Autodesk Fusion 360 part; units mm, degrees
(part 2 of 2)
extrude "Extrude1" add sketch "Sketch1" along normal blind 1.7 contours L0 L26 L52 L57 L77 L124 L128 L191 | L0 L12 L33 L120 L124 L128 L189 L191 | L0 L26 L33 L36 L52 L124 L128 L191 | L0 L12 L57 L120 L121 L124 L125 L128 L189 L191 | L0 L26 L57 L74 L76 L77 L191 L207 A39 | L0 L12 L57 L74 L121 L125 L126 L189 L191 L217 | L0 L12 L29 L32 L33 L189 L191 | L0 L26 L29 L33 L36 L191 | L26 L52 L57 L124 L127 L128 L220 | L26 L37 L52 L124 L128 L221 | L0 L26 L75 L78 L126 L191 L207 L217 L218 | L26 L75 L76 L78 L207 A39 | L26 L57 L76 L208 A39 | L0 L12 L28 L29 L32 A15 L189 L191 | L0 L26 L29 L36 A16 L191 | L26 L27 L33 L34 L36 L37 L39 L42 A26 L287 | L26 L27 L33 L34 A1 L36 L39 A26 | L52 L57 L123 L124 L127 | L0 L26 L122 L126 L191 L207 L218 | L0 L12 L121 L122 L126 L189 L191 | L26 L78 L207 A38 | L26 L76 L78 L207 L208 A38 A39 | L26 L76 L207 L208 A39 | L57 L127 L208 L219 L220 A39 | L3 L13 L26 L27 L30 L31 L35 L36 L39 A15 A16 L191 | L29 L30 A0 A1 | L26 L27 A1 L36 L39 A16 | L29 L30 A0 A1 | L27 L37 L39 L41 L42 L43 L287 L288 L289 L290 L291 L292 | L37 L41 L47 L52 L64 L109 L115 L119 L221 L288 | L52 L57 L123 L221 | L57 L123 L127 L208 L219 | L0 L26 L122 L130 L191 L193 L199 L207 | L0 L12 L122 L189 L191 L198 | L26 L78 L122 L123 A27 L207 A38 | L78 L126 A7 A38 L218 | L78 L126 A7 A38 L218 | L78 L127 A7 A38 L219 | L26 L27 L36 L39 A16 | L29 L30 A0 | L29 L30 A0 | L3 L27 L30 L34 L39 | L3 L27 L30 L39 A16 | L37 L40 L41 L44 L289 L293 | L3 L27 L34 L39 L43 L45 A25 L290 | L52 L57 L82 L114 L178 L221 | L57 L79 L123 L208 L221 | L78 L127 A7 A38 L219 | L78 L123 L208 A38 | L0 L12 L189 L191 L196 L197 L198 L199 | L25 L26 L78 L80 L83 L122 L123 L130 L131 A27 A28 L206 L207 L223 L224 L226 L230 L234 L237 | L78 L126 L127 A7 L218 L219 | L78 L126 L127 A7 L218 L219 | L78 L127 A7 L219 | L3 L13 L30 L34 L35 | L27 L37 L39 L40 L44 L45 L46 L47 L293 L294 L295 | L40 L44 L289 L291 L292 L293 L295 | L27 L39 L40 L43 L44 L289 L295 | L52 L57 L114 L115 L118 L212 | L57 L79 L81 L82 L208 L221 | L78 L79 L123 L208 L221 | L78 L127 A7 L219 | L0 L12 L189 L191 L193 L194 L195 L196 L197 L199 L200 | L25 L26 L130 L131 A9 A28 L206 L207 | L0 L26 L130 L134 L191 L207 | L3 L4 L13 L18 L19 L27 L34 L39 A24 A25 | L24 L27 L37 L38 L39 L46 L63 L64 L66 A23 A25 | L40 L44 L293 L294 L295 | L52 L57 L108 L115 L118 L119 L204 L212 | L57 L91 L114 L177 L208 L211 | L57 L91 L114 L118 L208 L211 L212 L216 | L57 L81 L179 L208 | L78 L79 L80 L81 L208 L221 | L0 L12 L130 L189 L191 L194 L200 | L25 L26 A9 A18 L206 L207 | L0 L26 L134 A18 L191 L207 | L134 L135 A8 A9 | L134 L135 A8 A9 | L0 L12 L129 L130 L134 L189 L191 | L24 L37 L38 L63 L64 A3 A23 | L37 L52 L60 L64 L181 | L52 L57 L108 L109 L110 L112 L115 L116 L119 | L57 L118 L208 L212 A36 | L57 L177 L178 L179 L208 | L78 L91 L114 L118 A6 L208 L211 L215 L216 | L78 L91 L114 L177 L208 L211 L215 | L78 L81 L86 L179 L208 | L25 L26 A18 L206 L207 | L21 L26 A18 L191 L207 | L0 L11 L12 L20 L129 L133 L134 A17 L189 L191 | L134 L135 A8 | L134 L135 A8 | L1 L25 L135 A18 L206 | L1 L25 L131 L135 L206 | L24 L27 L38 L39 A25 | L24 L37 L38 A3 A22 | L59 L60 A2 A3 L181 L184 | L37 L52 L60 L181 L182 A22 | L59 L60 A2 A3 L181 L184 | L52 L57 L64 L110 L112 L116 | L52 L57 L60 L64 L65 | L57 L108 L201 L202 L203 L204 | L57 L78 L108 L110 L112 L116 L201 | L57 L203 L208 A36 | L78 L118 A6 A37 | L78 L205 L208 A36 A37 | L78 L86 L177 L179 L208 | L78 L85 L91 L114 L170 L176 L177 L211 L215 | L78 L91 L113 L114 L117 A6 A29 L205 L210 L211 L213 L214 L215 | L78 L83 L86 L138 L139 L161 L164 L179 L222 L223 L238 L241 L250 | L20 L21 L22 L23 L191 | L1 L8 L15 L22 L23 L25 L132 L135 L136 A17 A18 L191 L206 | L1 L25 L131 L206 L230 | L1 L15 L131 L132 L135 | L4 L7 A24 | L16 L17 L18 L19 | L2 L7 L14 L16 L17 L24 L38 L71 A24 A25 | L2 L24 L38 L69 L70 A25 | L24 L37 L38 A22 | L24 L37 L48 L52 A22 | L59 L60 A2 L181 L184 | L59 L60 A2 L181 L184 | L24 L52 L57 L60 L61 L65 A21 L182 | L2 L24 L38 L59 L183 L184 A22 | L2 L24 L38 L59 L63 L184 | L108 L202 L205 A36 | L205 L208 A36 | L78 L118 A6 | L78 L118 A6 | L78 L117 A6 A37 | L78 L205 A37 | L78 L85 L86 L138 L176 L177 L179 L180 A32 L254 | L78 L117 L118 A6 | L91 A29 L210 L211 L214 L215 | L25 L83 L84 L206 L222 L223 L225 A44 L247 L248 A46 | L25 L83 L206 L223 L224 L225 L231 L232 A42 A47 A48 | L25 L206 L224 L225 L226 L227 L228 L229 A40 L230 | L1 L25 L206 L225 L229 L230 L232 L233 | L1 L15 L88 L92 L102 L131 L144 L154 L160 L233 L249 | L2 L24 L38 L66 L67 L69 | L2 L24 L48 L49 L50 L51 L52 | L2 L24 L38 L51 A22 | L2 L24 L38 L63 L67 | L2 L14 L50 L56 L58 L59 L62 A21 L183 | L2 L14 L59 L62 L63 | L78 L108 L110 L112 L116 L117 L209 | L78 L108 L117 L205 L209 | L78 L205 A36 | L78 L117 L118 A6 | L108 L113 L117 L205 L209 L210 L213 | L85 L91 L137 L165 L169 L170 L171 L172 L173 L176 L177 L251 | L85 L138 L168 L169 L176 L177 L180 A32 L254 | L91 L101 L113 L171 L173 L188 L205 L210 L214 | L25 L84 L85 L137 L138 L139 L140 L142 L143 L158 L159 A14 L180 A30 A34 L206 L250 L252 L253 L283 L284 L285 L286 A63 A64 A65 | L1 L25 L84 L206 L225 L232 L248 | L239 L240 A43 A44 | L222 L223 L238 L241 A44 | L239 L240 A43 A44 | L223 L224 L234 L237 A42 | L235 L236 A41 A42 | L235 L236 A41 A42 | L8 L11 A17 L191 | L25 L206 L224 L225 L227 L228 A40 L230 L231 L232 A47 A48 | L2 L14 L67 L68 L69 L73 | L2 L14 L69 L70 L71 L72 L73 | L2 L24 L49 L52 L53 A21 | L2 L14 L63 L67 | L108 L110 L112 L113 L117 L209 | L101 L108 L113 L205 L210 | L85 L137 L138 L165 L168 L169 L180 L251 L254 A66 | L138 L175 L180 A32 L253 L254 L280 L286 | L138 L139 L161 L164 A14 | L162 L163 A12 A14 | L162 L163 A12 A14 | L25 L84 L157 L206 L222 L225 L243 L244 A45 L246 L247 L248 A46 | L1 L25 L84 L155 L157 L206 L225 L245 L246 L248 L249 | L239 L240 A43 | L239 L240 A43 | L235 L236 A41 | L235 L236 A41 | L227 L228 A40 | L227 L228 A40 | L1 L15 L92 L93 L95 L102 L103 L106 | L2 L53 L56 A21 | L101 L108 L110 L113 | L101 A5 A31 L205 | L101 L105 L108 L205 | L85 L91 L137 L172 L173 L174 L251 | L166 L167 A13 A66 | L85 L137 L138 L174 L175 L180 A32 A33 L251 L254 L280 L281 L283 A66 | L166 L167 A13 A66 | L175 A33 L252 L253 L271 L272 L273 L274 L275 L278 L279 L280 L281 L282 L283 L286 A61 A62 | L252 L253 L275 L276 L277 L278 L279 L282 L283 L284 L285 L286 A56 A57 A59 A63 A64 A65 | L162 L163 A12 | L162 L163 A12 | L25 L84 L157 L206 L222 L225 L242 L243 L244 L245 A45 L246 | L139 A35 L222 L246 L250 | L1 L15 L93 L95 L98 L103 L106 L107 A19 | L1 L25 L89 L91 L95 L102 L106 L141 L206 | L1 L25 L87 L88 L89 L90 L91 L102 L141 L144 L206 | L100 L101 L105 L108 L110 | L91 L101 L102 L141 L185 L188 A31 | A5 L187 A31 | A5 L186 L187 A31 | L105 L106 A4 A5 | L25 A5 A20 L205 L206 | L105 A4 A5 A31 | L105 L108 A20 L205 | L85 L91 L137 L142 L174 L251 | L85 L137 L174 A33 L251 L252 L281 L283 | L166 L167 A13 | L166 L167 A13 | L253 L264 L270 L271 L278 L279 A61 | L252 L253 L267 L268 L269 L270 L275 L276 L277 L278 L279 L282 A54 A55 A56 A57 A58 A59 | L175 L280 A62 | L139 A35 L250 | L25 L84 L139 L149 L156 L157 A35 L206 L222 L242 L246 | L1 L25 L84 L140 L152 L153 L154 L155 L156 L157 L160 L206 L246 | L243 L244 A45 | L243 L244 A45 | L1 L25 L95 L106 A20 L206 | L1 L25 L84 L87 L140 L143 L144 L148 L206 | L25 L91 L102 A5 L141 A31 L206 | L25 L85 L90 L91 L102 L137 L141 L142 L145 L185 L206 | L25 L95 L97 A19 A20 L206 | L25 L100 L104 L105 L108 L110 A19 A20 L205 | A5 L186 L187 | A4 A5 L186 L187 A31 | A5 L186 A31 | L105 L106 A4 | L105 L106 A4 A31 | L106 A4 A5 A31 | L25 A20 L205 L206 | L175 L280 L281 A62 | L252 L253 L256 L257 L259 L262 L263 L264 L265 L266 L267 L270 L279 L282 A60 | L252 L253 L259 L260 L261 L262 L263 L266 L267 L268 L269 L270 L279 L282 A50 A51 A52 A54 A55 A58 | L175 A33 L281 L283 A62 | L25 L84 L139 L140 L150 L151 A11 L158 L159 A34 A35 L206 L250 | L25 L84 L139 L140 L149 L150 L151 L152 A11 L156 L206 | L1 L25 L84 L140 L153 L159 L160 L206 | L95 L97 L98 A19 | L1 L25 L84 L140 L143 L159 L206 | L25 L84 L85 L137 L140 L145 L146 L147 L148 A10 L206 | L25 L84 L85 L137 L140 L142 L143 L146 L147 A10 A30 L206 | A4 A31 | L252 L253 A49 L255 L256 L257 L258 L259 L262 L263 L266 L279 L282 A53 | L252 L253 A49 L255 L258 L259 L260 L261 L262 L263 L266 L279 L282 A50 A51 A52 | L264 L265 A60 | L271 L274 A61 | L271 L272 L273 L274 A61 | L252 L265 L267 L274 L275 L282 A61 | L252 L253 A49 L255 L258 L263 L266 L279 L282 | L252 L253 A49 L255 L258 L263 L266 L279 L282 | L256 L257 A53 | L150 L151 A11 | L150 L151 A11 | L146 L147 A10 | L146 L147 A10 makes body 1
extrude "Extrude2" add sketch "Sketch1" along normal blind 13.7 contours L0 L12 L33 L120 L124 L128 L189 L191 | L0 L12 L57 L120 L121 L124 L125 L128 L189 L191 | L0 L12 L57 L74 L121 L125 L126 L189 L191 L217 | L0 L12 L29 L32 L33 L189 L191 | L0 L12 L28 L29 L32 A15 L189 L191 | L0 L12 L121 L122 L126 L189 L191 | L3 L13 L26 L27 L30 L31 L35 L36 L39 A15 A16 L191 | L0 L12 L122 L189 L191 L198 | L26 L27 L36 L39 A16 | L0 L12 L189 L191 L196 L197 L198 L199 | L3 L13 L30 L34 L35 | L0 L12 L189 L191 L193 L194 L195 L196 L197 L199 L200 | L3 L4 L13 L18 L19 L27 L34 L39 A24 A25 | L0 L12 L130 L189 L191 L194 L200 | L0 L12 L129 L130 L134 L189 L191 | L52 L57 L108 L109 L110 L112 L115 L116 L119 | L25 L26 A18 L206 L207 | L21 L26 A18 L191 L207 | L0 L11 L12 L20 L129 L133 L134 A17 L189 L191 | L24 L27 L38 L39 A25 | L52 L57 L64 L110 L112 L116 | L52 L57 L60 L64 L65 | L57 L78 L108 L110 L112 L116 L201 | L20 L21 L22 L23 L191 | L1 L8 L15 L22 L23 L25 L132 L135 L136 A17 A18 L191 L206 | L1 L15 L131 L132 L135 | L4 L7 A24 | L16 L17 L18 L19 | L2 L7 L14 L16 L17 L24 L38 L71 A24 A25 | L24 L37 L38 A22 | L24 L37 L48 L52 A22 | L24 L52 L57 L60 L61 L65 A21 L182 | L1 L15 L88 L92 L102 L131 L144 L154 L160 L233 L249 | L2 L24 L48 L49 L50 L51 L52 | L2 L24 L38 L51 A22 | L2 L14 L50 L56 L58 L59 L62 A21 L183 | L2 L14 L59 L62 L63 | L78 L108 L110 L112 L116 L117 L209 | L8 L11 A17 L191 | L2 L14 L67 L68 L69 L73 | L2 L14 L69 L70 L71 L72 L73 | L2 L24 L49 L52 L53 A21 | L2 L14 L63 L67 | L108 L110 L112 L113 L117 L209 | L1 L15 L92 L93 L95 L102 L103 L106 | L2 L53 L56 A21 | L101 L108 L110 L113 | L1 L15 L93 L95 L98 L103 L106 L107 A19 | L100 L101 L105 L108 L110 | L25 L95 L97 A19 A20 L206 | L25 L100 L104 L105 L108 L110 A19 A20 L205 | L25 A20 L205 L206 | L95 L97 L98 A19 bodies 1
extrude "Extrude3" add sketch "Sketch1" along normal up to surface (13.7 mm away) contours L0 L26 L52 L57 L77 L124 L128 L191 | L0 L12 L57 L120 L121 L124 L125 L128 L189 L191 | L26 L52 L57 L124 L127 L128 L220 | L52 L57 L123 L124 L127 | L52 L57 L123 L221 | L52 L57 L82 L114 L178 L221 | L52 L57 L114 L115 L118 L212 | L52 L57 L108 L115 L118 L119 L204 L212 | L52 L57 L108 L109 L110 L112 L115 L116 L119 bodies 1
extrude "Extrude4" add sketch "Sketch1" along normal up to surface (13.7 mm away) contours L0 L26 L57 L74 L76 L77 L191 L207 A39 | L26 L57 L76 L208 A39 | L26 L76 L207 L208 A39 | L57 L108 L201 L202 L203 L204 | L57 L203 L208 A36 | L108 L202 L205 A36 | L205 L208 A36 bodies 1
extrude "Extrude5" cut sketch "Sketch1" against normal blind 2 from surface at 13.7 contours L0 L12 L189 L191 L196 L197 L198 L199 | L0 L12 L189 L191 L193 L194 L195 L196 L197 L199 L200 | L2 L14 L67 L68 L69 L73 | L2 L14 L69 L70 L71 L72 L73 bodies 1
extrude "Extrude6" add 1 faces at (60.9667, -0.5667, 11.7) along direction (0, 0, 1) blind 0.5 on bodies 1 bodies 1
extrude "Extrude7" add sketch "Sketch1" along normal blind 7 from surface at 1.7 contours L85 L91 L137 L165 L169 L170 L171 L172 L173 L176 L177 L251 | L85 L138 L168 L169 L176 L177 L180 A32 L254 | L85 L137 L138 L165 L168 L169 L180 L251 L254 A66 | L162 L163 A12 A14 | L162 L163 A12 A14 | L85 L91 L137 L172 L173 L174 L251 | L166 L167 A13 A66 | L85 L137 L138 L174 L175 L180 A32 A33 L251 L254 L280 L281 L283 A66 | L166 L167 A13 A66 | L1 L25 L87 L88 L89 L90 L91 L102 L141 L144 L206 | L91 L101 L102 L141 L185 L188 A31 | L25 L84 L139 L149 L156 L157 A35 L206 L222 L242 L246 | L1 L25 L84 L140 L152 L153 L154 L155 L156 L157 L160 L206 L246 | L1 L25 L84 L87 L140 L143 L144 L148 L206 | L25 L85 L90 L91 L102 L137 L141 L142 L145 L185 L206 | L175 L280 L281 A62 | L175 A33 L281 L283 A62 | L25 L84 L139 L140 L150 L151 A11 L158 L159 A34 A35 L206 L250 | L25 L84 L139 L140 L149 L150 L151 L152 A11 L156 L206 | L1 L25 L84 L140 L153 L159 L160 L206 | L25 L84 L85 L137 L140 L145 L146 L147 L148 A10 L206 | L25 L84 L85 L137 L140 L142 L143 L146 L147 A10 A30 L206 bodies 1
extrude "Extrude8" add sketch "Sketch1" along normal blind 11 from surface at 1.7 contours L1 L25 L84 L206 L225 L232 L248 | L1 L25 L84 L155 L157 L206 L225 L245 L246 L248 L249 | L1 L25 L84 L140 L152 L153 L154 L155 L156 L157 L160 L206 L246 bodies 1
extrude "Extrude9" cut sketch "Sketch1" along normal blind 20 from surface at 1.7 contours L52 L57 L123 L221 bodies 1
extrude "Extrude10" cut 2 faces at (120.5, 52.5, 12.7) (120.5, 52.5, 12.7) along direction (0, 0, 1) up to surface end surface through (0, 0, 1.7) normal (0, 0, 1) offset 0 on bodies 1 bodies 1
extrude "Extrude11" add sketch "Sketch1" along normal up to surface (8.7 mm away) contours L25 L206 L224 L225 L226 L227 L228 L229 A40 L230 | L1 L25 L206 L225 L229 L230 L232 L233 | L239 L240 A43 A44 | L239 L240 A43 A44 | L235 L236 A41 A42 | L235 L236 A41 A42 | L25 L206 L224 L225 L227 L228 A40 L230 L231 L232 A47 A48 | L25 L84 L157 L206 L222 L225 L243 L244 A45 L246 L247 L248 A46 | L1 L25 L84 L155 L157 L206 L225 L245 L246 L248 L249 | L25 L84 L157 L206 L222 L225 L242 L243 L244 L245 A45 L246 | L139 A35 L222 L246 L250 | L139 A35 L250 | L1 L25 L84 L140 L152 L153 L154 L155 L156 L157 L160 L206 L246 | L1 L25 L84 L140 L153 L159 L160 L206 bodies 1
extrude "Extrude12" add sketch "Sketch1" along normal blind 26.3 from surface at 1.7 contours L0 L26 L75 L78 L126 L191 L207 L217 L218 | L26 L75 L76 L78 L207 A39 | L0 L26 L122 L126 L191 L207 L218 | L26 L76 L78 L207 L208 A38 A39 | L57 L127 L208 L219 L220 A39 | L57 L123 L127 L208 L219 | L26 L78 L122 L123 A27 L207 A38 | L78 L126 A7 A38 L218 | L78 L126 A7 A38 L218 | L78 L127 A7 A38 L219 | L78 L127 A7 A38 L219 | L78 L123 L208 A38 | L25 L26 L130 L131 A9 A28 L206 L207 | L0 L26 L130 L134 L191 L207 | L57 L91 L114 L118 L208 L211 L212 L216 | L25 L26 A9 A18 L206 L207 | L0 L26 L134 A18 L191 L207 | L134 L135 A8 A9 | L134 L135 A8 A9 | L57 L118 L208 L212 A36 | L78 L91 L114 L118 A6 L208 L211 L215 L216 | L1 L25 L135 A18 L206 | L1 L25 L131 L135 L206 | L78 L118 A6 A37 | L78 L205 L208 A36 A37 | L78 L91 L113 L114 L117 A6 A29 L205 L210 L211 L213 L214 L215 | L78 L117 A6 A37 | L78 L205 A37 | L78 L108 L117 L205 L209 | L78 L205 A36 | L108 L113 L117 L205 L209 L210 L213 | L101 A5 A31 L205 | L101 L105 L108 L205 | L1 L25 L89 L91 L95 L102 L106 L141 L206 | A5 L187 A31 | A5 L186 L187 A31 | L105 L106 A4 A5 | L25 A5 A20 L205 L206 | L105 A4 A5 A31 | L105 L108 A20 L205 | L1 L25 L95 L106 A20 L206 | L25 L91 L102 A5 L141 A31 L206 | A5 L186 L187 | A4 A5 L186 L187 A31 | A5 L186 A31 | L106 A4 A5 A31 bodies 1
extrude "Extrude13" add sketch "Sketch1" along normal blind 30 contours L0 L26 L57 L74 L76 L77 L191 L207 A39 | L0 L12 L57 L74 L121 L125 L126 L189 L191 L217 | L26 L57 L76 L208 A39 | L0 L12 L121 L122 L126 L189 L191 | L26 L76 L207 L208 A39 | L0 L12 L122 L189 L191 L198 | L0 L12 L189 L191 L196 L197 L198 L199 | L0 L12 L189 L191 L193 L194 L195 L196 L197 L199 L200 | L0 L12 L130 L189 L191 L194 L200 | L0 L12 L129 L130 L134 L189 L191 | L25 L26 A18 L206 L207 | L21 L26 A18 L191 L207 | L0 L11 L12 L20 L129 L133 L134 A17 L189 L191 | L57 L108 L201 L202 L203 L204 | L57 L78 L108 L110 L112 L116 L201 | L57 L203 L208 A36 | L20 L21 L22 L23 L191 | L1 L8 L15 L22 L23 L25 L132 L135 L136 A17 A18 L191 L206 | L1 L15 L131 L132 L135 | L108 L202 L205 A36 | L205 L208 A36 | L1 L15 L88 L92 L102 L131 L144 L154 L160 L233 L249 | L78 L108 L110 L112 L116 L117 L209 | L8 L11 A17 L191 | L108 L110 L112 L113 L117 L209 | L1 L15 L92 L93 L95 L102 L103 L106 | L101 L108 L110 L113 | L1 L15 L93 L95 L98 L103 L106 L107 A19 | L100 L101 L105 L108 L110 | L25 L95 L97 A19 A20 L206 | L25 L100 L104 L105 L108 L110 A19 A20 L205 | L25 A20 L205 L206 | L95 L97 L98 A19 bodies 1
extrude "Extrude14" cut sketch "Sketch1" along normal blind 1.5 from surface at 13.7 contours L0 L12 L189 L191 L196 L197 L198 L199 | L0 L12 L189 L191 L193 L194 L195 L196 L197 L199 L200 bodies 1
extrude "Extrude15" cut 1 faces at (60.9667, -0.5667, 13.7) along direction (0, 0, -1) blind 1.5 on bodies 1 bodies 1
extrude "Extrude16" add 2 faces at (36.1667, 118.4333, 13.7) (-1.1333, 132.3333, 13.7) along direction (0, 0, 1) blind 5.3 on bodies 1 bodies 1
extrude "Extrude17" add 1 faces at (18.8, 201.1333, 11.7) along direction (0, 0, 1) blind 5.3 on bodies 1 bodies 1
extrude "Extrude18" add sketch "Sketch1" along normal blind 5.3 from surface at 1.7 contours L0 L26 L33 L36 L52 L124 L128 L191 | L0 L26 L29 L33 L36 L191 | L26 L37 L52 L124 L128 L221 | L0 L26 L29 L36 A16 L191 | L26 L27 L33 L34 L36 L37 L39 L42 A26 L287 | L26 L27 L33 L34 A1 L36 L39 A26 | L29 L30 A0 A1 | L26 L27 A1 L36 L39 A16 | L29 L30 A0 A1 | L27 L37 L39 L41 L42 L43 L287 L288 L289 L290 L291 L292 | L37 L41 L47 L52 L64 L109 L115 L119 L221 L288 | L29 L30 A0 | L29 L30 A0 | L3 L27 L30 L34 L39 | L3 L27 L30 L39 A16 | L37 L40 L41 L44 L289 L293 | L3 L27 L34 L39 L43 L45 A25 L290 | L27 L37 L39 L40 L44 L45 L46 L47 L293 L294 L295 | L40 L44 L289 L291 L292 L293 L295 | L27 L39 L40 L43 L44 L289 L295 | L24 L27 L37 L38 L39 L46 L63 L64 L66 A23 A25 | L40 L44 L293 L294 L295 | L24 L37 L38 L63 L64 A3 A23 | L37 L52 L60 L64 L181 | L24 L37 L38 A3 A22 | L59 L60 A2 A3 L181 L184 | L37 L52 L60 L181 L182 A22 | L59 L60 A2 A3 L181 L184 | L2 L24 L38 L69 L70 A25 | L59 L60 A2 L181 L184 | L59 L60 A2 L181 L184 | L2 L24 L38 L59 L183 L184 A22 | L2 L24 L38 L59 L63 L184 | L2 L24 L38 L66 L67 L69 | L2 L24 L38 L63 L67 bodies 1
extrude "Extrude19" cut 1 faces at (11.8667, 76.3333, 7) along direction (0, 0, -1) blind 2 on bodies 1 bodies 1
extrude "Extrude20" cut 1 faces at (18.8, 201.1333, 17) along direction (0, 0, -1) blind 2 on bodies 1 bodies 1
extrude "Extrude21" cut 2 faces at (36.1667, 118.4333, 19) (-1.1333, 132.3333, 19) along direction (0, 0, -1) blind 2 on bodies 1 bodies 1
extrude "Extrude22" add sketch "Sketch1" along normal blind 24 contours L0 L26 L29 L33 L36 L191 | L0 L26 L29 L36 A16 L191 | L26 L27 L33 L34 A1 L36 L39 A26 | L29 L30 A0 A1 | L26 L27 A1 L36 L39 A16 | L29 L30 A0 A1 | L3 L27 L30 L34 L39 | L3 L27 L30 L39 A16 | L24 L37 L38 L63 L64 A3 A23 | L37 L52 L60 L64 L181 | L24 L37 L38 A3 A22 | L59 L60 A2 A3 L181 L184 | L37 L52 L60 L181 L182 A22 | L59 L60 A2 A3 L181 L184 | L2 L24 L38 L59 L183 L184 A22 | L2 L24 L38 L59 L63 L184 bodies 1
extrude "Extrude23" add sketch "Sketch1" against normal blind 2 from surface at 30 separate body contours L0 L26 L52 L57 L77 L124 L128 L191 | L0 L12 L33 L120 L124 L128 L189 L191 | L0 L26 L33 L36 L52 L124 L128 L191 | L0 L12 L57 L120 L121 L124 L125 L128 L189 L191 | L0 L12 L29 L32 L33 L189 L191 | L0 L26 L29 L33 L36 L191 | L26 L52 L57 L124 L127 L128 L220 | L26 L37 L52 L124 L128 L221 | L0 L12 L28 L29 L32 A15 L189 L191 | L0 L26 L29 L36 A16 L191 | L26 L27 L33 L34 L36 L37 L39 L42 A26 L287 | L26 L27 L33 L34 A1 L36 L39 A26 | L52 L57 L123 L124 L127 | L3 L13 L26 L27 L30 L31 L35 L36 L39 A15 A16 L191 | L29 L30 A0 A1 | L26 L27 A1 L36 L39 A16 | L29 L30 A0 A1 | L27 L37 L39 L41 L42 L43 L287 L288 L289 L290 L291 L292 | L37 L41 L47 L52 L64 L109 L115 L119 L221 L288 | L52 L57 L123 L221 | L26 L27 L36 L39 A16 | L3 L27 L30 L34 L39 | L3 L27 L30 L39 A16 | L37 L40 L41 L44 L289 L293 | L3 L27 L34 L39 L43 L45 A25 L290 | L52 L57 L82 L114 L178 L221 | L3 L13 L30 L34 L35 | L27 L37 L39 L40 L44 L45 L46 L47 L293 L294 L295 | L40 L44 L289 L291 L292 L293 L295 | L27 L39 L40 L43 L44 L289 L295 | L52 L57 L114 L115 L118 L212 | L3 L4 L13 L18 L19 L27 L34 L39 A24 A25 | L24 L27 L37 L38 L39 L46 L63 L64 L66 A23 A25 | L40 L44 L293 L294 L295 | L52 L57 L108 L115 L118 L119 L204 L212 | L24 L37 L38 L63 L64 A3 A23 | L37 L52 L60 L64 L181 | L52 L57 L108 L109 L110 L112 L115 L116 L119 | L24 L27 L38 L39 A25 | L24 L37 L38 A3 A22 | L59 L60 A2 A3 L181 L184 | L37 L52 L60 L181 L182 A22 | L59 L60 A2 A3 L181 L184 | L52 L57 L64 L110 L112 L116 | L52 L57 L60 L64 L65 | L4 L7 A24 | L16 L17 L18 L19 | L2 L7 L14 L16 L17 L24 L38 L71 A24 A25 | L2 L24 L38 L69 L70 A25 | L24 L37 L38 A22 | L24 L37 L48 L52 A22 | L24 L52 L57 L60 L61 L65 A21 L182 | L2 L24 L38 L59 L183 L184 A22 | L2 L24 L38 L59 L63 L184 | L2 L24 L38 L66 L67 L69 | L2 L24 L48 L49 L50 L51 L52 | L2 L24 L38 L51 A22 | L2 L24 L38 L63 L67 | L2 L14 L50 L56 L58 L59 L62 A21 L183 | L2 L14 L59 L62 L63 | L2 L14 L67 L68 L69 L73 | L2 L14 L69 L70 L71 L72 L73 | L2 L24 L49 L52 L53 A21 | L2 L14 L63 L67 | L2 L53 L56 A21 makes body 2
extrude "Extrude24" add sketch "Sketch1" against normal blind 4 from surface at 28 contours L0 L26 L29 L33 L36 L191 | L0 L26 L29 L36 A16 L191 | L26 L27 L33 L34 A1 L36 L39 A26 | L29 L30 A0 A1 | L26 L27 A1 L36 L39 A16 | L29 L30 A0 A1 | L3 L27 L30 L34 L39 | L3 L27 L30 L39 A16 | L24 L37 L38 L63 L64 A3 A23 | L37 L52 L60 L64 L181 | L24 L37 L38 A3 A22 | L59 L60 A2 A3 L181 L184 | L37 L52 L60 L181 L182 A22 | L59 L60 A2 A3 L181 L184 | L2 L24 L38 L59 L183 L184 A22 | L2 L24 L38 L59 L63 L184 bodies 2
extrude "Extrude25" add sketch "Sketch1" against normal blind 11 from surface at 28 contours L0 L26 L52 L57 L77 L124 L128 L191 | L0 L12 L33 L120 L124 L128 L189 L191 | L0 L12 L57 L120 L121 L124 L125 L128 L189 L191 | L0 L12 L29 L32 L33 L189 L191 | L26 L52 L57 L124 L127 L128 L220 | L0 L12 L28 L29 L32 A15 L189 L191 | L52 L57 L123 L124 L127 | L3 L13 L26 L27 L30 L31 L35 L36 L39 A15 A16 L191 | L52 L57 L123 L221 | L26 L27 L36 L39 A16 | L52 L57 L82 L114 L178 L221 | L3 L13 L30 L34 L35 | L52 L57 L114 L115 L118 L212 | L3 L4 L13 L18 L19 L27 L34 L39 A24 A25 | L52 L57 L108 L115 L118 L119 L204 L212 | L52 L57 L108 L109 L110 L112 L115 L116 L119 | L24 L27 L38 L39 A25 | L52 L57 L64 L110 L112 L116 | L52 L57 L60 L64 L65 | L4 L7 A24 | L16 L17 L18 L19 | L2 L7 L14 L16 L17 L24 L38 L71 A24 A25 | L24 L37 L38 A22 | L24 L37 L48 L52 A22 | L24 L52 L57 L60 L61 L65 A21 L182 | L2 L24 L48 L49 L50 L51 L52 | L2 L24 L38 L51 A22 | L2 L14 L50 L56 L58 L59 L62 A21 L183 | L2 L14 L59 L62 L63 | L2 L14 L67 L68 L69 L73 | L2 L14 L69 L70 L71 L72 L73 | L2 L24 L49 L52 L53 A21 | L2 L14 L63 L67 | L2 L53 L56 A21 bodies 2
extrude "Extrude26" cut sketch "Sketch1" along normal blind 2 from surface at 17 contours L2 L14 L67 L68 L69 L73 | L2 L14 L69 L70 L71 L72 L73 bodies 2
extrude "Extrude27" cut sketch "Sketch1" against normal blind 2 from surface at 30 contours L29 L30 A0 A1 | L29 L30 A0 A1 | L59 L60 A2 A3 L181 L184 | L59 L60 A2 A3 L181 L184 bodies 2
extrude "Extrude28" add sketch "Sketch1" against normal blind 2 from surface at 30 separate body contours L26 L78 L207 A38 | L26 L78 L122 L123 A27 L207 A38 | L78 L126 A7 A38 L218 | L78 L126 A7 A38 L218 | L78 L127 A7 A38 L219 | L78 L127 A7 A38 L219 | L78 L123 L208 A38 | L25 L26 L78 L80 L83 L122 L123 L130 L131 A27 A28 L206 L207 L223 L224 L226 L230 L234 L237 | L78 L79 L123 L208 L221 | L25 L26 L130 L131 A9 A28 L206 L207 | L78 L79 L80 L81 L208 L221 | L134 L135 A8 A9 | L134 L135 A8 A9 | L78 L91 L114 L118 A6 L208 L211 L215 L216 | L78 L91 L114 L177 L208 L211 L215 | L78 L81 L86 L179 L208 | L78 L118 A6 A37 | L78 L86 L177 L179 L208 | L78 L85 L91 L114 L170 L176 L177 L211 L215 | L78 L91 L113 L114 L117 A6 A29 L205 L210 L211 L213 L214 L215 | L78 L83 L86 L138 L139 L161 L164 L179 L222 L223 L238 L241 L250 | L78 L117 A6 A37 | L78 L85 L86 L138 L176 L177 L179 L180 A32 L254 | L91 A29 L210 L211 L214 L215 | L25 L83 L84 L206 L222 L223 L225 A44 L247 L248 A46 | L25 L83 L206 L223 L224 L225 L231 L232 A42 A47 A48 | L25 L206 L224 L225 L226 L227 L228 L229 A40 L230 | L85 L91 L137 L165 L169 L170 L171 L172 L173 L176 L177 L251 | L85 L138 L168 L169 L176 L177 L180 A32 L254 | L91 L101 L113 L171 L173 L188 L205 L210 L214 | L25 L84 L85 L137 L138 L139 L140 L142 L143 L158 L159 A14 L180 A30 A34 L206 L250 L252 L253 L283 L284 L285 L286 A63 A64 A65 | L239 L240 A43 A44 | L222 L223 L238 L241 A44 | L239 L240 A43 A44 | L223 L224 L234 L237 A42 | L235 L236 A41 A42 | L235 L236 A41 A42 | L25 L206 L224 L225 L227 L228 A40 L230 L231 L232 A47 A48 | L85 L137 L138 L165 L168 L169 L180 L251 L254 A66 | L138 L175 L180 A32 L253 L254 L280 L286 | L138 L139 L161 L164 A14 | L162 L163 A12 A14 | L162 L163 A12 A14 | L25 L84 L157 L206 L222 L225 L243 L244 A45 L246 L247 L248 A46 | L239 L240 A43 | L239 L240 A43 | L235 L236 A41 | L235 L236 A41 | L227 L228 A40 | L227 L228 A40 | L101 A5 A31 L205 | L85 L91 L137 L172 L173 L174 L251 | L166 L167 A13 A66 | L85 L137 L138 L174 L175 L180 A32 A33 L251 L254 L280 L281 L283 A66 | L166 L167 A13 A66 | L175 A33 L252 L253 L271 L272 L273 L274 L275 L278 L279 L280 L281 L282 L283 L286 A61 A62 | L252 L253 L275 L276 L277 L278 L279 L282 L283 L284 L285 L286 A56 A57 A59 A63 A64 A65 | L162 L163 A12 | L162 L163 A12 | L25 L84 L157 L206 L222 L225 L242 L243 L244 L245 A45 L246 | L139 A35 L222 L246 L250 | L91 L101 L102 L141 L185 L188 A31 | A5 L187 A31 | A5 L186 L187 A31 | L105 L106 A4 A5 | L105 A4 A5 A31 | L85 L91 L137 L142 L174 L251 | L85 L137 L174 A33 L251 L252 L281 L283 | L166 L167 A13 | L166 L167 A13 | L175 L280 A62 | L139 A35 L250 | L25 L84 L139 L149 L156 L157 A35 L206 L222 L242 L246 | L243 L244 A45 | L243 L244 A45 | L25 L91 L102 A5 L141 A31 L206 | L25 L85 L90 L91 L102 L137 L141 L142 L145 L185 L206 | A5 L186 L187 | A4 A5 L186 L187 A31 | A5 L186 A31 | L106 A4 A5 A31 | L175 L280 L281 A62 | L175 A33 L281 L283 A62 | L25 L84 L139 L140 L150 L151 A11 L158 L159 A34 A35 L206 L250 | L25 L84 L139 L140 L149 L150 L151 L152 A11 L156 L206 | L25 L84 L85 L137 L140 L145 L146 L147 L148 A10 L206 | L25 L84 L85 L137 L140 L142 L143 L146 L147 A10 A30 L206 | L271 L272 L273 L274 A61 | L150 L151 A11 | L150 L151 A11 | L146 L147 A10 | L146 L147 A10 makes body 3
extrude "Extrude29" add 1 faces at (74.6333, 127.1, 8.7) along direction (0, 0, -1) up to surface (7 mm away) on bodies 1 bodies 1
extrude "Extrude30" cut 1 faces at (74.6333, 127.1, 8.7) along direction (0, 0, -1) blind 6 on bodies 1 bodies 1
extrude "Extrude31" add 1 faces at (74.6333, 127.1, 2.7) along direction (0, 0, -1) blind 1 on bodies 1 bodies 1
extrude "Extrude32" add sketch "Sketch1" along normal blind 7 from surface at 1.7 contours L166 L167 A13 A66 | L166 L167 A13 A66 bodies 1
extrude "Extrude33" cut 1 faces at (72.3498, 123.6685, 2.7) along direction (0, 0, -1) blind 1 on bodies 1 bodies 1
extrude "Extrude34" add sketch "Sketch1" against normal blind 1 from surface at 28 separate body contours L175 A33 L252 L253 L271 L272 L273 L274 L275 L278 L279 L280 L281 L282 L283 L286 A61 A62 | L252 L253 L275 L276 L277 L278 L279 L282 L283 L284 L285 L286 A56 A57 A59 A63 A64 A65 | L253 L264 L270 L271 L278 L279 A61 | L252 L253 L267 L268 L269 L270 L275 L276 L277 L278 L279 L282 A54 A55 A56 A57 A58 A59 | L252 L253 L256 L257 L259 L262 L263 L264 L265 L266 L267 L270 L279 L282 A60 | L252 L253 L259 L260 L261 L262 L263 L266 L267 L268 L269 L270 L279 L282 A50 A51 A52 A54 A55 A58 | L175 A33 L281 L283 A62 | L252 L253 A49 L255 L256 L257 L258 L259 L262 L263 L266 L279 L282 A53 | L252 L253 A49 L255 L258 L259 L260 L261 L262 L263 L266 L279 L282 A50 A51 A52 | L264 L265 A60 | L271 L274 A61 | L271 L272 L273 L274 A61 | L252 L265 L267 L274 L275 L282 A61 | L252 L253 A49 L255 L258 L263 L266 L279 L282 | L252 L253 A49 L255 L258 L263 L266 L279 L282 | L256 L257 A53 makes body 4
extrude "Extrude35" cut sketch "Sketch1" along normal blind 30 contours L252 L253 A49 L255 L258 L263 L266 L279 L282 | L252 L253 A49 L255 L258 L263 L266 L279 L282 bodies 4
extrude "Extrude36" add sketch "Sketch1" along normal blind 3 from surface at 28 contours L252 L253 L256 L257 L259 L262 L263 L264 L265 L266 L267 L270 L279 L282 A60 | L252 L253 L259 L260 L261 L262 L263 L266 L267 L268 L269 L270 L279 L282 A50 A51 A52 A54 A55 A58 | L252 L253 A49 L255 L256 L257 L258 L259 L262 L263 L266 L279 L282 A53 | L252 L253 A49 L255 L258 L259 L260 L261 L262 L263 L266 L279 L282 A50 A51 A52 | L252 L253 A49 L255 L258 L263 L266 L279 L282 | L252 L253 A49 L255 L258 L263 L266 L279 L282 | L256 L257 A53 bodies 4
extrude "Extrude37" add sketch "Sketch1" against normal blind 5 from surface at 27 contours L252 L253 A49 L255 L256 L257 L258 L259 L262 L263 L266 L279 L282 A53 | L252 L253 A49 L255 L258 L259 L260 L261 L262 L263 L266 L279 L282 A50 A51 A52 bodies 4
extrude "Extrude38" cut sketch "Sketch1" along normal blind 55 contours L40 L44 L289 L291 L292 L293 L295 | L40 L44 L293 L294 L295 bodies 2
named bodies: "akrilik"
